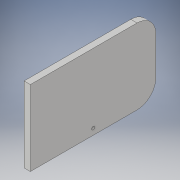
# Autodesk Inventor part: Part1
Saved by Autodesk Inventor 2018.2 (Build 222227000, 227)
## iProperties
Created: 2018-02-01
Part Number: Part1
Material: Generic
Document SubType Name: Modeling
Designer: MIABo
Density: 1 g/cm^3
Appearance: Default
Author: MIABo
Autodesk Inventor part; units mm, degrees
ref_plane "YZ Plane" through (0, 0, 0) normal (1, 0, 0) x (0, 1, 0)
ref_plane "XZ Plane" through (0, 0, 0) normal (0, 1, 0) x (-1, 0, 0)
ref_plane "XY Plane" through (0, 0, 0) normal (0, 0, 1) x (1, 0, 0)
sketch "Sketch1" plane through (0, 0, 0) normal (1, 0, 0) x (0, 1, 0)
  line L0 (100.5124, 128.0095) -> (100.5124, -87.8905)
  line L1 (62.4124, -125.9905) -> (-13.7876, -125.9905)
  line L2 (-51.8876, -87.8905) -> (-51.8876, 128.0095)
  line L3 (-51.8876, 128.0095) -> (100.5124, 128.0095)
  arc A0 (62.4124, -125.9905) -> (100.5124, -87.8905) centre (62.4124, -87.8905) ccw
  arc A1 (-51.8876, -87.8905) -> (-13.7876, -125.9905) centre (-13.7876, -87.8905) ccw
  point P0 (0, 0)
  point P1 (100.5124, -125.9905)
  dimension "d0" = 254
  dimension "d1" = 152.4
  dimension "d3" = 38.1
  constraints: 8 end point, 4 point on circle, 4 tangent, 3 perpendicular, 2 centre point, 2 point on line, 1 vertical
  measures "d0" distance of L0.start point (100.512, -125.991)
  measures "d1" distance of L2.end L0.start
  measures "d3" radius of A1
extrude "Extrusion1" add sketch "Sketch1" along normal blind 12.7
sketch "Sketch3" plane through (12.7, 0, 0) normal (1, 0, 0) x (0, 0, -1)
  line L0 (125.9905, -13.7876) -> (125.9905, 62.4124) projected
  line L1 (-128.0095, 100.5124) -> (-128.0095, -51.8876) projected
  line L2 (-128.0095, -51.8876) -> (87.8905, -51.8876) projected
  point P0 (0, 0)
  point P1 (-1.0095, -39.1876)
  dimension "d16" = 254
  dimension "d17" = 127
  dimension "d18" = 12.7
  measures "d16" distance between parallel lines of L0 L1
  measures "d17" distance from line of L1 point (-1.009, -39.188)
  measures "d18" distance from line of L2 point (-1.009, -39.188)
hole "Hole2" at (12.7, -39.1876, 1.0095) direction (-1, 0, 0) diameter 6.35 end through all
body "Solid1"
